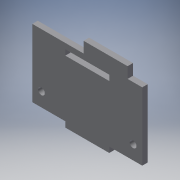
# Autodesk Inventor part: Pan base top side bars
Saved by Autodesk Inventor 2018 (Build 220112000, 112)
## iProperties
Created: 2018-06-25
Part Number: Pan base top side bars
Material: Generic
Document SubType Name: Modeling
Designer: Ajith Thomas
Density: 1 g/cm^3
Appearance: Default
Author: Ajith Thomas
Autodesk Inventor part; units mm, degrees
ref_plane "YZ Plane" through (0, 0, 0) normal (1, 0, 0) x (0, 1, 0)
ref_plane "XZ Plane" through (0, 0, 0) normal (0, 1, 0) x (-1, 0, 0)
ref_plane "XY Plane" through (0, 0, 0) normal (0, 0, 1) x (1, 0, 0)
sketch "Sketch1" plane through (0, 0, 0) normal (0, 0, 1) x (1, 0, 0)
  line L0 (42, 0) -> (60, 0) projected
  line L1 (42, 0) -> (18, 0) projected
  line L2 (0, 0) -> (18, 0) projected
  line L3 (60, 0) -> (60, 3) construction
  line L4 (0, 0) -> (0, 3) construction
  line L5 (24, 16) -> (47, 16) construction
  line L6 (60, 0) -> (0, 0)
  line L7 (0, 0) -> (0, 40)
  line L8 (0, 40) -> (60, 40)
  line L9 (60, 40) -> (60, 0)
  line L10 (52, 40) -> (28, 40)
  line L11 (28, 40) -> (28, 46)
  line L12 (28, 46) -> (52, 46)
  line L13 (52, 46) -> (52, 40)
  line L14 (42, 3) -> (42, 0) construction
  line L15 (18, 0) -> (18, 3) construction
  line L16 (42, 34) -> (18, 34)
  line L17 (18, 34) -> (18, 37)
  line L18 (18, 37) -> (42, 37)
  line L19 (42, 37) -> (42, 34)
  dimension "d0" = 40
  dimension "d1" = 8
  dimension "d2" = 24
  dimension "d3" = 6
  dimension "d4" = 3
  dimension "d5" = 3
  dimension "d6" = 24
  constraints: 24 end point, 6 parallel, 3 horizontal, 3 perpendicular, 1 point on line
  measures "d0" distance of L6.end L7.end
  measures "d1" distance between parallel lines of L9 L13
  measures "d2" distance between parallel lines of L11 L13
  measures "d3" distance between parallel lines of L8 L12
  measures "d4" distance between parallel lines of L8 L18
  measures "d5" distance between parallel lines of L18 L16
  measures "d6" distance between parallel lines of L17 L19
extrude "Extrusion1" add sketch "Sketch1" against normal blind 3
sketch "Sketch2" plane through (0, 0, 0) normal (0, 0, 1) x (1, 0, 0)
  line L0 (42, 0) -> (42, 3) projected
  line L1 (60, 3) -> (42, 3) projected
  line L2 (60, 0) -> (60, 3) projected
  line L3 (60, 0) -> (42, 0) projected
  line L4 (18, 3) -> (18, 0) projected
  line L5 (18, 0) -> (0, 0) projected
  line L6 (0, 0) -> (0, 3) projected
  line L7 (18, 3) -> (0, 3) projected
extrude "Extrusion2" cut sketch "Sketch2" against normal blind 3
sketch "Sketch3" plane through (0, 0, -3) normal (0, 0, -1) x (-1, 0, 0)
  arc A0 (-3.15, 12.05) -> (-6.85, 12.05) centre (-5, 12.05) ccw construction
  line L0 (-3.15, 12.05) -> (-3.15, 9.25) construction
  arc A1 (-6.85, 9.25) -> (-3.15, 9.25) centre (-5, 9.25) ccw construction
  line L1 (-6.85, 9.25) -> (-6.85, 12.05) construction
  arc A2 (-9, 17.6) -> (-10, 16.6) centre (-9, 16.6) ccw construction
  line L2 (-10, 16.6) -> (-10, 4) construction
  line L3 (-10, 4) -> (0, 4) construction
  line L4 (0, 4) -> (0, 16.6) construction
  arc A3 (0, 16.6) -> (-1, 17.6) centre (-1, 16.6) ccw construction
  line L5 (-1, 17.6) -> (-9, 17.6) construction
  arc A4 (-53.15, 12.05) -> (-56.85, 12.05) centre (-55, 12.05) ccw construction
  line L6 (-53.15, 12.05) -> (-53.15, 9.25) construction
  arc A5 (-56.85, 9.25) -> (-53.15, 9.25) centre (-55, 9.25) ccw construction
  line L7 (-56.85, 9.25) -> (-56.85, 12.05) construction
  arc A6 (-59, 17.6) -> (-60, 16.6) centre (-59, 16.6) ccw construction
  line L8 (-60, 16.6) -> (-60, 4) construction
  line L9 (-60, 4) -> (-50, 4) construction
  line L10 (-50, 4) -> (-50, 16.6) construction
  arc A7 (-50, 16.6) -> (-51, 17.6) centre (-51, 16.6) ccw construction
  line L11 (-51, 17.6) -> (-59, 17.6) construction
  line L12 (-5, 9.25) -> (-5, 12.05) construction
  line L13 (-55, 9.25) -> (-55, 12.05) construction
  circle A8 centre (-5, 10.65) radius 1.85
  circle A9 centre (-55, 10.65) radius 1.85
  point P0 (0, 0)
  constraints: 4 end point, 2 centre point, 2 midpoint, 2 tangent, 2 vertical
extrude "Extrusion3" cut sketch "Sketch3" against normal blind 22.4
body "Solid1"
